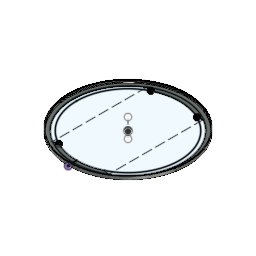
cardboard_spool_ring (Autodesk Fusion 360 design; units mm, degrees)
Autodesk Fusion 360 part; units mm, degrees
sketch "Ring" plane through (0, 0, 0) normal (1, 0, 0) x (0, 1, 0)
  line L0 (0, 0) -> (0, 5.5)
  line L1 (0, 0) -> (14, 0)
  line L2 (14, 0) -> (14, 1)
  line L3 (14, 1) -> (1, 1)
  line L4 (1, 1) -> (1, 4)
  line L5 (1, 4) -> (1.5, 4.5)
  line L6 (1.5, 4.5) -> (1.5, 5.5)
  line L7 (0, 5.5) -> (1.5, 5.5)
  line L8 (101, -11) -> (101, 21) construction
  point P0 (101, 0)
  dimension "d11" = 1
  dimension "d12" = 3
  dimension "d13" = 1
  dimension "d21" = 1
  dimension "d44" = 135
  dimension "d45" = 0.5
  dimension "d47" = 13
  dimension "d48" = 100
  constraint coincident L0.start L1.start
  constraint vertical L0
  constraint perpendicular L0 L1
  constraint perpendicular L1 L2
  constraint perpendicular L2 L3
  constraint perpendicular L3 L4
  constraint vertical L6
  constraint horizontal L7
  constraint vertical L8
  constraint coincident P0 L8
  measures "d11" distance of L1.end L2.end
  measures "d12" distance of L3.end L4.end
  measures "d13" distance of L5.end L6.end
  measures "d21" distance of L0 L4
  measures "d44" angle of L4 L5
  measures "d45" distance of L4 L6
  measures "d47" distance of L2.end L3.end
  measures "d48" distance of L4 L8
revolve "Revolve Ring" add sketch "Ring" angle 360 about axis through (0, 101, -11) along (0, 0, 1)
sketch "Cutout" plane through (0, 0, 1) normal (0, 0, 1) x (-1, 0, 0)
  circle A0 centre (0, -101) radius 100
  circle A1 centre (0, -101) radius 87
  circle A2 centre (0, -101) radius 87
  circle A3 centre (0, -101) radius 93
  line L0 (39.1124, -23.2876) -> (47.8845, -21.275)
  line L1 (-38.6062, -23.0349) -> (-47.365, -20.9653)
  line L2 (-38.6062, -178.9651) -> (-47.365, -181.0347)
  line L3 (39.1124, -178.7124) -> (47.8845, -180.725)
  line L4 (47.8845, -180.725) -> (47.8845, -21.275) construction
  line L5 (-47.365, -181.0347) -> (-47.365, -20.9653) construction
  point P0 (39.1124, -23.2876)
  dimension "d24" = 0
  dimension "d25" = 186
  dimension "d37" = 9
  dimension "d49" = 95.25
  dimension "d50" = 77.719
  dimension "d52" = 159.45
  constraint coincident A1 P0
  constraint concentric A0 A3
  constraint coincident A1 L3.start
  constraint coincident A1 L2.start
  constraint coincident A2 L1.start
  constraint coincident P0 L0.start
  constraint coincident A3 L0.end
  constraint coincident A3 L1.end
  constraint coincident A3 L2.end
  constraint coincident A3 L3.end
  constraint parallel L4 L5
  constraint vertical L5
  constraint equal L0 L1
  constraint equal L1 L2
  constraint equal L2 L3
  measures "d25" diameter of A3
  measures "d37" distance of L3.start L3.end
  measures "d49" distance of L2.end L3.end
  measures "d50" distance of L3.start L2.start
  measures "d52" distance of L0.end L3.end
extrude "Remove Cutout" cut sketch "Cutout" against normal blind 10 contours A1 A2 A3 L0 L3 | A1 A2 A3 L1 L2
fillet "Fillet2" radius 1 1 edges at (-93.2327, 64.8385, 1)
equation "d11 = bottom_thickness"
equation "d12 = cardboard_thickness"
equation "d21 = edge_thickness"
equation "d25 = spool_diameter - ( 2 * width_to_holes )"
equation "bottom_thickness = 1 mm" comment "Thickness of the part that touches the spool on the side."
equation "cardboard_thickness = 3 mm" comment "Thickness of the cardboard on the spool."
equation "spool_diameter = 200 mm" comment "Diameter of the spool."
equation "edge_thickness = 1 mm" comment "Thickness of the part that goes around the edge of the cardboard spool and sits on the rollers in the AMS, adding to the diameter of the spool.  Decrease this if the AMS cannot be closed as the diameter is too big.  For example: If the spool diameter is 200 mm and this value is 1 mm, the final diameter of the printed spool ring will be 200 mm + (2 * 1 mm) = 202 mm (as there is material on both sides)."
equation "width_to_holes = 7 mm" comment "Width between the edge of the cardboard spool and right before the holes start (which you use to stick the loose end of the filement in for storage). Decrease this if the printed part covers holes on the cardboard spool."
equation "total_width = 13 mm" comment "Width of the printed part that covers the cardboard spool's side (one side only). Must be larger than or equal to \"width_to_holes\"."
equation "d47 = total_width"
equation "d48 = spool_diameter / 2"
equation "fillet_radius = 1 mm" comment "Size of the internal fillet, to increase strength in case the layers separate when taking it off the bed."
named bodies: "Ring"
